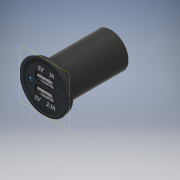
# Autodesk Inventor part: usb_outlet
Saved by Autodesk Inventor 2019.2 (Build 232265000, 265)
## iProperties
Created: 2020-05-18
Part Number: usb_outlet
Material: Thermoplastic Resin
Document SubType Name: Modeling
Designer: Johansson
Density: 1.28 g/cm^3
Appearance: Smooth - Black
Author: Johansson
Autodesk Inventor part; units mm, degrees
ref_plane "YZ Plane" through (0, 0, 0) normal (1, 0, 0) x (0, 1, 0)
ref_plane "XZ Plane" through (0, 0, 0) normal (0, 1, 0) x (-1, 0, 0)
ref_plane "XY Plane" through (0, 0, 0) normal (0, 0, 1) x (1, 0, 0)
sketch "Sketch1" plane through (0, 0, 0) normal (0, 0, 1) x (1, 0, 0)
  circle A0 centre (0, 0) radius 14.5
  dimension "d0" = 29
  constraints: 1 centre point, 1 coincident
  measures "d0" diameter of A0
extrude "Extrusion1" add sketch "Sketch1" along normal blind 51
sketch "Sketch2" plane through (0, 0, 51) normal (0, 0, 1) x (1, 0, 0)
  circle A0 centre (0, 0) radius 19.5
  circle A1 centre (0, 0) radius 14.5 projected
  dimension "d3" = 5
  constraints: 1 centre point, 1 coincident
  measures "d3" radial gap between concentric circles of A1 A0
extrude "Extrusion2" add sketch "Sketch2" along normal blind 3 contours A0 | A1
sketch "Sketch3" plane through (0, 0, 54) normal (0, 0, 1) x (1, 0, 0)
  line L0 (-21.7015, 20.032) -> (19.2808, 20.032) construction
  line L1 (19.2808, 20.032) -> (19.2808, -20.9503) construction
  line L2 (19.2808, -20.9503) -> (-21.7015, -20.9503) construction
  line L3 (-21.7015, -20.9503) -> (-21.7015, 20.032) construction
  constraints: 2 other
equation "\"d0\" = r_usboutlet"
equation "\"wl_panel\" = 265"
equation "\"t_panel\" = 8"
equation "\"r_button\" = 8"
equation "\"l_stereo\" = 178"
equation "\"d_stereo\" = 177"
equation "\"w_label\" = 15"
equation "\"r_labelscrew\" = 2.5"
equation "\"ro_labelscrew\" = 5"
equation "\"l_buttontobutton\" = 25"
equation "\"r_usboutlet\" = 29"
equation "\"l_fastener_button\" = 19"
body "Solid1"
